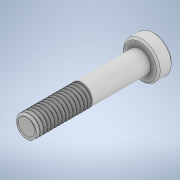
# Autodesk Inventor part: bolt
Saved by Autodesk Inventor 2022.1 (Build 261234000, 234)
## iProperties
Created: 2020-10-19
Part Number: bolt
Material: Generic
Document SubType Name: Modeling
Designer: dwbertol
Density: 1 g/cm^3
Appearance: Default
Author: dwbertol
## iProperties of the stored document _3DPrint.ipt
Created: 2020-10-19
Part Number: _3DPrint
Material: Generic
Document SubType Name: Modeling
Designer: dwbertol
Density: 1 g/cm^3
Appearance: Default
Author: dwbertol
Autodesk Inventor part; units mm, degrees
ref_plane "YZ Plane" through (0, 0, 0) normal (1, 0, 0) x (0, 1, 0)
ref_plane "XZ Plane" through (0, 0, 0) normal (0, 1, 0) x (-1, 0, 0)
ref_plane "XY Plane" through (0, 0, 0) normal (0, 0, 1) x (1, 0, 0)
sketch "Sketch1" plane through (0, 0, 0) normal (0, 0, 1) x (1, 0, 0)
  circle A0 centre (0, 0) radius 5
  dimension "d0" = 10
  constraints: 1 centre point, 1 coincident
  measures "d0" diameter of A0
extrude "Extrusion1" add sketch "Sketch1" along normal blind 4
sketch "Sketch2" plane through (0, 0, 4) normal (0, 0, 1) x (1, 0, 0)
  circle A0 centre (0, 0) radius 2.95
  dimension "d3" = 5.9
  constraints: 1 centre point, 1 coincident
  measures "d3" diameter of A0
extrude "Extrusion2" add sketch "Sketch2" along normal blind 31
chamfer "Chamfer2" distance 0.5 angle 45 2 edges at (-5, 0, 0) (-5, 0, 4)
sketch "Sketch4" plane through (0, 0, 0) normal (0, 0, -1) x (-1, 0, 0)
  line L0 (-0.6, 2.25) -> (0.6, 2.25)
  line L1 (0.6, 2.25) -> (0.6, -2.25)
  line L2 (0.6, -2.25) -> (-0.6, -2.25)
  line L3 (-0.6, -2.25) -> (-0.6, 2.25)
  line L4 (-0.6, 0) -> (0.6, 0) construction
  line L5 (0, 2.25) -> (0, -2.25) construction
  point P0 (0, 0)
  dimension "d24" = 1.2
  dimension "d25" = 4.5
  constraints: 12 end point, 6 midpoint, 2 parallel, 1 horizontal, 1 perpendicular
  measures "d24" distance between parallel lines of L1 L3
  measures "d25" distance from line of L5.start L2
extrude "Extrusion3" cut sketch "Sketch4" against normal blind 3
thread "Thread6" size "M6x1" class "6g" standard "ANSI Metric M Profile" length 15
sketch "Sketch18" plane through (0, 0, 35) normal (-1, 0, 0) x (0, 1, 0)
  line L0 (2.95, 0) -> (2.95, 15)
  line L1 (2.95, 15) -> (2.2085, 15)
  line L2 (2.2085, 15) -> (2.2085, 0)
  line L3 (2.2085, 0) -> (2.95, 0)
  line L4 (0, -8.3086) -> (0, 42.2181) projected
  constraints: 8 end point
revolve "Revolution8" cut sketch "Sketch18" angle 360 about axis through (0, 0, 35) along (0, 0, -1)
sketch "Sketch19" plane through (0, 0, 35) normal (-1, 0, 0) x (0, 1, 0)
  line L0 (2.95, 0) -> (2.95, 15)
  line L1 (2.95, 15) -> (2.2085, 15)
  line L2 (2.2085, 15) -> (2.2085, 0)
  line L3 (2.2085, 0) -> (2.95, 0)
  line L4 (0, -8.3086) -> (0, 42.2181) projected
  constraints: 8 end point
revolve "Revolution9" add sketch "Sketch19" angle 360 about axis through (0, 0, 35) along (0, 0, -1) separate body
sketch "Sketch17" plane through (0, 0, 35) normal (1, 0, 0) x (0, 0, -1)
  line L0 (-0.5834, -2.2593) -> (-0.5001, -2.2593) construction
  line L1 (0.0832, -2.8996) -> (-0.0001, -3.0597) construction
  line L2 (-1.0001, -3.0597) -> (-1.0834, -2.8996) construction
  line L3 (-0.4168, -2.2593) -> (-0.5001, -2.0992) construction
  line L4 (-0.5001, -2.0992) -> (-0.5834, -2.2593) construction
  line L5 (-1.0001, -3.0597) -> (-0.9168, -2.8996) construction
  line L6 (-0.4168, -2.2593) -> (-0.0834, -2.8996)
  line L7 (-1.0834, -2.8996) -> (-0.9168, -2.8996) construction
  arc A0 (-1.0834, -2.8996) -> (-1.0001, -2.9502) centre (-1.0001, -2.8562) ccw construction
  line L8 (0.0832, -2.8996) -> (-0.0834, -2.8996) construction
  line L9 (-1.0001, -3.0597) -> (-1.0001, -2.8996) construction
  line L10 (-0.0001, -3.0597) -> (-0.0001, -2.8996) construction
  line L11 (-0.5001, -2.0992) -> (-0.5001, -2.2087) construction
  line L12 (-1.0001, -2.9502) -> (-0.0001, -2.9502)
  arc A1 (-1.0001, -2.9502) -> (-0.9168, -2.8996) centre (-1.0001, -2.8562) ccw
  line L13 (-0.0834, -2.8996) -> (-0.0001, -3.0597) construction
  line L14 (-0.9168, -2.8996) -> (-0.5834, -2.2593)
  line L15 (-0.0001, -0.0002) -> (-0.0001, 0.0177)
  line L16 (-0.0001, 0.0177) -> (-0.0001, -0.0002)
  line L17 (-0.0001, -0.0002) -> (0.0334, -0.0002)
  arc A2 (-0.0834, -2.8996) -> (-0.0001, -2.9502) centre (-0.0001, -2.8562) ccw
  arc A3 (-0.0001, -2.9502) -> (0.0832, -2.8996) centre (-0.0001, -2.8562) ccw construction
  arc A4 (-0.5001, -2.2087) -> (-0.5834, -2.2593) centre (-0.5001, -2.3027) ccw
  arc A5 (-0.4168, -2.2593) -> (-0.5001, -2.2087) centre (-0.5001, -2.3027) ccw
  line L18 (-0.5001, -2.2087) -> (-0.5001, -2.2593) construction
  line L19 (-0.5001, -2.2593) -> (-0.4168, -2.2593) construction
  dimension "d104" = 55
  dimension "d105" = 0.1601
  dimension "d106" = 0.1601
  dimension "Sketch17_ThreadOffset" = 0
  dimension "Sketch17_MajorRadius" = 2.95
  dimension "d109" = 1
  dimension "Sketch17_MinorRadius" = 2.2085
  constraints: 40 end point, 12 point on circle, 10 parallel, 8 tangent, 6 centre point, 6 collinear, 2 midpoint, 2 point on line, 1 horizontal, 1 perpendicular, 3 other
  measures "d104" angle of L6 L14
  measures "d105" distance of L3.end L0.end
  measures "d106" distance of L1.end L10.end
  measures "Sketch17_ThreadOffset" distance between parallel lines of L15 L10
  measures "Sketch17_MajorRadius" distance from line of L12 L15.start
  measures "d109" distance from line of L1.end L9
  measures "Sketch17_MinorRadius" distance edge to line of A5 L17
coil "Coil5" sketch "Sketch17" operation cut axis through (0, 0, 35) along (0, 0, -1) pitch 1.001 turns 16.983017 hand right bodies 2
equation "\"d104\" = d111"
equation "\"d105\" = 0.160083 * Sketch17_Pitch"
equation "\"d106\" = 0.160083 * Sketch17_Pitch"
equation "\"d109\" = Sketch17_Pitch"
equation "\"d43\" = 55deg"
equation "\"Sketch7_Pitch\" = 0.7"
equation "\"d67\" = 55deg"
equation "\"Sketch11_Pitch\" = 1"
equation "\"d90\" = 55deg"
equation "\"Sketch14_Pitch\" = 1"
equation "\"d111\" = 55deg"
equation "\"Sketch17_Pitch\" = 1"
body "Solid1"
body "Solid5"
